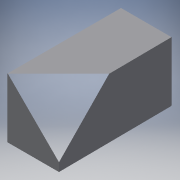
# Autodesk Inventor part: Guide
Saved by Autodesk Inventor 2016 (Build 200138000, 138)
## iProperties
Created: 2017-06-08
Part Number: Guide
Material: Generic
Document SubType Name: Modeling
Designer: Owner
Density: 1 g/cm^3
Appearance: Default
Author: Owner
Autodesk Inventor part; units mm, degrees
ref_plane "YZ Plane" through (0, 0, 0) normal (1, 0, 0) x (0, 1, 0)
ref_plane "XZ Plane" through (0, 0, 0) normal (0, 1, 0) x (-1, 0, 0)
ref_plane "XY Plane" through (0, 0, 0) normal (0, 0, 1) x (1, 0, 0)
sketch "Sketch1" plane through (0, 0, 0) normal (0, 0, 1) x (1, 0, 0)
  line L0 (-20.9848, 52.6481) -> (-30.7638, 52.6481) projected
  line L1 (-30.7638, 20.8981) -> (-30.7638, 52.6481) projected
  line L2 (-20.9848, 20.8981) -> (-30.7638, 20.8981) projected
  line L3 (-20.9848, 52.6481) -> (-20.9848, 20.8981) projected
  line L4 (-22.6993, 26.2773) -> (-22.6993, 24.127) projected
  line L5 (-22.6993, 24.127) -> (-29.0493, 24.127) projected
  line L6 (-29.0493, 24.127) -> (-29.0493, 26.2773) projected
  line L7 (-29.0493, 26.2773) -> (-22.6993, 26.2773) projected
  line L8 (-22.6993, 32.7351) -> (-22.6993, 30.5848) projected
  line L9 (-22.6993, 30.5848) -> (-29.0493, 30.5848) projected
  line L10 (-29.0493, 30.5848) -> (-29.0493, 32.7351) projected
  line L11 (-29.0493, 32.7351) -> (-22.6993, 32.7351) projected
  line L12 (-22.6993, 39.1928) -> (-22.6993, 37.0425) projected
  line L13 (-22.6993, 37.0425) -> (-29.0493, 37.0425) projected
  line L14 (-29.0493, 37.0425) -> (-29.0493, 39.1928) projected
  line L15 (-29.0493, 39.1928) -> (-22.6993, 39.1928) projected
  line L16 (-22.6993, 45.6505) -> (-22.6993, 43.5002) projected
  line L17 (-22.6993, 43.5002) -> (-29.0493, 43.5002) projected
  line L18 (-29.0493, 43.5002) -> (-29.0493, 45.6505) projected
  line L19 (-29.0493, 45.6505) -> (-22.6993, 45.6505) projected
  line L20 (-22.6993, 52.1083) -> (-22.6993, 49.958) projected
  line L21 (-22.6993, 49.958) -> (-29.0493, 49.958) projected
  line L22 (-29.0493, 49.958) -> (-29.0493, 52.1083) projected
  line L23 (-29.0493, 52.1083) -> (-22.6993, 52.1083) projected
  line L24 (-22.6993, 48.8794) -> (-22.6993, 46.7291) projected
  line L25 (-22.6993, 46.7291) -> (-29.0493, 46.7291) projected
  line L26 (-29.0493, 46.7291) -> (-29.0493, 48.8794) projected
  line L27 (-29.0493, 48.8794) -> (-22.6993, 48.8794) projected
  line L28 (-22.6993, 42.4217) -> (-22.6993, 40.2714) projected
  line L29 (-22.6993, 40.2714) -> (-29.0493, 40.2714) projected
  line L30 (-29.0493, 40.2714) -> (-29.0493, 42.4217) projected
  line L31 (-29.0493, 42.4217) -> (-22.6993, 42.4217) projected
  line L32 (-22.6993, 35.9639) -> (-22.6993, 33.8136) projected
  line L33 (-22.6993, 33.8136) -> (-29.0493, 33.8136) projected
  line L34 (-29.0493, 33.8136) -> (-29.0493, 35.9639) projected
  line L35 (-29.0493, 35.9639) -> (-22.6993, 35.9639) projected
  line L36 (-22.6993, 29.5062) -> (-22.6993, 27.3559) projected
  line L37 (-22.6993, 27.3559) -> (-29.0493, 27.3559) projected
  line L38 (-29.0493, 27.3559) -> (-29.0493, 29.5062) projected
  line L39 (-29.0493, 29.5062) -> (-22.6993, 29.5062) projected
  line L40 (-22.6993, 23.0485) -> (-22.6993, 20.8982) projected
  line L41 (-22.6993, 20.8982) -> (-29.0493, 20.8982) projected
  line L42 (-29.0493, 20.8982) -> (-29.0493, 23.0485) projected
  line L43 (-29.0493, 23.0485) -> (-22.6993, 23.0485) projected
  line L44 (-20.9848, 20.8981) -> (-20.4848, 20.8981)
  line L45 (-20.4848, 20.8981) -> (-30.7638, 20.8981)
  line L46 (-30.7638, 20.8981) -> (-31.2638, 20.8981)
  line L47 (-30.7638, 20.8981) -> (-30.7638, 24.7081) projected
  line L48 (-30.8638, 52.6481) -> (-20.7348, 52.6481)
  line L49 (-20.7348, 52.6481) -> (-20.4848, 24.7081)
  line L50 (-20.4848, 24.7081) -> (-30.8638, 24.7081)
  line L51 (-30.8638, 24.7081) -> (-31.2638, 24.7081)
  line L52 (-31.2638, 24.7081) -> (-31.2638, 52.6481)
  line L53 (-31.2638, 52.6481) -> (-20.7348, 52.6481)
  point P0 (0, 0)
  dimension "d0" = 0.5
  dimension "d1" = 0.5
  constraints: 18 end point, 3 perpendicular, 2 horizontal, 1 collinear, 1 point on line
  measures "d0" distance of L2.start L44.end
  measures "d1" distance of L1.start L46.end
extrude "Extrusion1" add sketch "Sketch1" along normal blind 12.41 contours L3 L50 L4 L7 L6 L1 L0 | L48 L49 L50 L3 | L1 L50 L51 L52 L53 L48 | L50 L6 L7 L4 | L8 L9 L10 L11 | L12 L13 L14 L15 | L16 L17 L18 L19 | L20 L21 L22 L23 | L24 L25 L26 L27 | L28 L29 L30 L31 | L32 L33 L34 L35 | L36 L37 L38 L39
sketch "Sketch2" plane through (-31.2638, 24.7081, 0) normal (-1, 0, 0) x (0, 0, 1)
  line L0 (12.41, 1.27) -> (22.57, 1.27) projected
  line L1 (12.41, 1.27) -> (0, 1.27)
  line L2 (0, 1.27) -> (0, 4.27)
  line L3 (0, 4.27) -> (12.41, 4.27)
  line L4 (12.41, 4.27) -> (12.41, 1.27)
  line L5 (0, 0) -> (12.41, 0) projected
  line L6 (12.41, 0) -> (0, 0)
  line L7 (0, 0) -> (0, 1.27)
  line L8 (0, 1.27) -> (12.41, 1.27)
  line L9 (12.41, 1.27) -> (12.41, 0)
  point P0 (0, -24.7081)
  dimension "d4" = 3
  constraints: 16 end point, 4 parallel, 2 horizontal, 2 perpendicular
  measures "d4" distance between parallel lines of L1 L3
extrude "Extrusion2" cut sketch "Sketch2" against normal blind 12.41
sketch "Sketch3" plane through (-31.2638, 52.6481, 0) normal (-1, 0, 0) x (0, 0, 1)
  line L0 (25.999, 0) -> (12.41, 0) projected
  line L1 (12.41, -26.67) -> (12.41, 0) projected
  line L2 (12.41, -26.67) -> (22.57, -26.67) projected
  line L3 (22.57, -26.67) -> (22.57, -27.94) projected
  line L4 (22.57, -27.94) -> (12.41, -27.94) projected
  line L5 (12.41, -31.75) -> (12.41, -27.94) projected
  line L6 (25.999, -31.75) -> (12.41, -31.75) projected
  line L7 (25.999, -31.75) -> (25.999, 0) projected
  line L8 (0, -23.67) -> (12.41, -23.67) projected
  line L9 (12.41, 0) -> (12.41, -23.67) projected
  line L10 (0, 0) -> (12.41, 0) projected
  line L11 (0, 0) -> (0, -23.67) projected
  line L12 (0, 0) -> (25.999, 0)
  line L13 (25.999, 0) -> (25.999, -23.67)
  line L14 (25.999, -23.67) -> (0, -23.67)
  line L15 (0, -23.67) -> (0, 0)
  point P0 (0, -52.6481)
  constraints: 8 end point, 2 parallel, 1 horizontal, 1 perpendicular, 1 point on line
extrude "Extrusion3" add sketch "Sketch3" along normal blind 3 contours L7 L14 L1 L0 | L1 L8 L11 L10
sketch "Sketch4" plane through (-20.7348, 52.6481, 12.41) normal (1, 0.0089, 0) x (0, 0, -1)
  line L0 (0, -23.6709) -> (12.41, -23.6709) projected
  line L1 (12.41, -23.6709) -> (12.41, 0) projected
  line L2 (12.41, 0) -> (0, 0) projected
  line L3 (0, -23.6709) -> (0, 0) projected
  line L4 (0, 0.0022) -> (-13.589, 0.0022) projected
  line L5 (-13.589, 0.0022) -> (-13.589, -31.7465) projected
  line L6 (-13.589, -31.7465) -> (0, -31.7465) projected
  line L7 (0, -27.9366) -> (0, -31.7465) projected
  line L8 (0, -27.9366) -> (-10.16, -27.9366) projected
  line L9 (-10.16, -27.9366) -> (-10.16, -26.6667) projected
  line L10 (-10.16, -26.6667) -> (0, -26.6667) projected
  line L11 (0, 0.0022) -> (0, -26.6667) projected
  line L12 (0, -23.6709) -> (12.41, -23.6709) projected
  line L13 (-13.589, 0.0022) -> (12.41, 0.0022)
  line L14 (12.41, 0.0022) -> (12.41, -23.6709)
  line L15 (12.41, -23.6709) -> (-13.589, -23.6709)
  line L16 (-13.589, -23.6709) -> (-13.589, 0.0022)
  point P0 (12.41, -52.8315)
  constraints: 8 end point, 2 parallel, 1 horizontal, 1 perpendicular
extrude "Extrusion4" add sketch "Sketch4" along normal blind 3 contours L3 L2 L1 L0 | L15 L5 L4 L11 L3 | L11 L13 L14 L2
body "Solid1"
